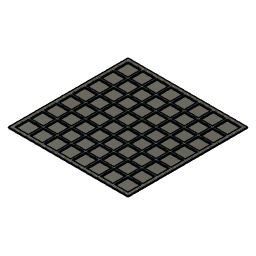
šachovnice v3 (Autodesk Fusion 360 design; units mm, degrees)
Autodesk Fusion 360 part; units mm, degrees
sketch "Sketch1" plane through (0, 0, 0) normal (0, 0, 1) x (1, 0, 0)
  line L0 (-133.2, 0) -> (133.2, 0)
  line L1 (133.2, 0) -> (133.2, -266.4)
  line L2 (133.2, -266.4) -> (-133.2, -266.4)
  line L3 (-133.2, -266.4) -> (-133.2, 0)
  line L4 (-100.2, 0) -> (-100.2, -266.4) construction
  line L5 (-133.2, -33.3) -> (133.2, -33.3) construction
  line L6 (-66.9, 0) -> (-66.9, -266.4) construction
  line L7 (-33.6, 0) -> (-33.6, -266.4) construction
  line L8 (-0.3, 0) -> (-0.3, -266.4) construction
  line L9 (33, 0) -> (33, -266.4) construction
  line L10 (66.3, 0) -> (66.3, -266.4) construction
  line L11 (99.6, 0) -> (99.6, -266.4) construction
  line L12 (-133.2, -66.6) -> (133.2, -66.6) construction
  line L13 (-133.2, -99.9) -> (133.2, -99.9) construction
  line L14 (-133.2, -133.2) -> (133.2, -133.2) construction
  line L15 (-133.2, -166.5) -> (133.2, -166.5) construction
  line L16 (-133.2, -199.8) -> (133.2, -199.8) construction
  line L17 (-133.2, -233.1) -> (133.2, -233.1) construction
  line L18 (-102.2, 0) -> (-102.2, -266.4)
  line L19 (-68.9, 0) -> (-68.9, -266.4)
  line L20 (-35.6, 0) -> (-35.6, -266.4)
  line L21 (-2.3, 0) -> (-2.3, -266.4)
  line L22 (31, 0) -> (31, -266.4)
  line L23 (64.3, 0) -> (64.3, -266.4)
  line L24 (97.6, 0) -> (97.6, -266.4)
  line L25 (-133.2, -35.3) -> (133.2, -35.3)
  line L26 (-133.2, -31.3) -> (133.2, -31.3)
  line L27 (-98.2, 0) -> (-98.2, -266.4)
  line L28 (-64.9, 0) -> (-64.9, -266.4)
  line L29 (-31.6, 0) -> (-31.6, -266.4)
  line L30 (1.7, 0) -> (1.7, -266.4)
  line L31 (35, 0) -> (35, -266.4)
  line L32 (68.3, 0) -> (68.3, -266.4)
  line L33 (101.6, 0) -> (101.6, -266.4)
  line L34 (-133.2, -64.6) -> (133.2, -64.6)
  line L35 (-133.2, -68.6) -> (133.2, -68.6)
  line L36 (-133.2, -97.9) -> (133.2, -97.9)
  line L37 (-133.2, -101.9) -> (133.2, -101.9)
  line L38 (-133.2, -131.2) -> (133.2, -131.2)
  line L39 (-133.2, -135.2) -> (133.2, -135.2)
  line L40 (-133.2, -164.5) -> (133.2, -164.5)
  line L41 (-133.2, -168.5) -> (133.2, -168.5)
  line L42 (-133.2, -197.8) -> (133.2, -197.8)
  line L43 (-133.2, -201.8) -> (133.2, -201.8)
  line L44 (-133.2, -231.1) -> (133.2, -231.1)
  line L45 (-133.2, -235.1) -> (133.2, -235.1)
  line L46 (137.2, -270.4) -> (-137.2, -270.4)
  line L47 (-137.2, -270.4) -> (-137.2, 4)
  line L48 (-137.2, 4) -> (137.2, 4)
  line L49 (137.2, 4) -> (137.2, -270.4)
  line L50 (-141.2, -274.4) -> (-141.2, 8)
  line L51 (-141.2, 8) -> (141.2, 8)
  line L52 (141.2, 8) -> (141.2, -274.4)
  line L53 (141.2, -274.4) -> (-141.2, -274.4)
  dimension "d1" = 266.4
  dimension "d8" = 33.3
  dimension "d9" = 0
  dimension "d10" = 33
  dimension "d11" = 33.3
  dimension "d14" = 0
  dimension "d15" = -33.3
  dimension "d16" = 2
  dimension "d17" = 2
  dimension "d18" = -2
  dimension "d19" = -2
  dimension "d20" = -4
  dimension "d21" = -8
  constraint horizontal L0
  constraint vertical L1
  constraint horizontal L2
  constraint vertical L3
  constraint equal L0 L3
  constraint midpoint origin L0
  constraint coincident L0 L4.start
  constraint coincident L2 L4.end
  constraint perpendicular L2 L4
  constraint coincident L3 L5.start
  constraint coincident L1 L5.end
  constraint perpendicular L1 L5
  measures "d1" distance of L0.start L0.end
  measures "d10" distance of L3 L4
  measures "d11" distance of L0 L5
extrude "Extrude1" add sketch "Sketch1" along normal blind 4 contours L0 L18 L26 L27 | L3 L18 L25 L26 | L18 L25 L26 L27 | L0 L19 L26 L28 | L19 L25 L26 L27 | L18 L25 L27 L34 | L3 L18 L34 L35 | L19 L25 L26 L28 | L18 L27 L34 L35 | L0 L20 L26 L29 | L20 L25 L26 L28 | L19 L25 L28 L34 | L19 L27 L34 L35 | L18 L27 L35 L36 | L3 L18 L36 L37 | L20 L25 L26 L29 | L19 L28 L34 L35 | L18 L27 L36 L37 | L0 L21 L26 L30 | L21 L25 L26 L29 | L20 L25 L29 L34 | L20 L28 L34 L35 | L19 L28 L35 L36 | L19 L27 L36 L37 | L18 L27 L37 L38 | L3 L18 L38 L39 | L21 L25 L26 L30 | L20 L29 L34 L35 | L19 L28 L36 L37 | L18 L27 L38 L39 | L0 L22 L26 L31 | L22 L25 L26 L30 | L21 L25 L30 L34 | L21 L29 L34 L35 | L20 L29 L35 L36 | L20 L28 L36 L37 | L19 L28 L37 L38 | L19 L27 L38 L39 | L18 L27 L39 L40 | L3 L18 L40 L41 | L22 L25 L26 L31 | L21 L30 L34 L35 | L20 L29 L36 L37 | L19 L28 L38 L39 | L18 L27 L40 L41 | L0 L23 L26 L32 | L23 L25 L26 L31 | L22 L25 L31 L34 | L22 L30 L34 L35 | L21 L30 L35 L36 | L21 L29 L36 L37 | L20 L29 L37 L38 | L20 L28 L38 L39 | L19 L28 L39 L40 | L19 L27 L40 L41 | L18 L27 L41 L42 | L3 L18 L42 L43 | L23 L25 L26 L32 | L22 L31 L34 L35 | L21 L30 L36 L37 | L20 L29 L38 L39 | L19 L28 L40 L41 | L18 L27 L42 L43 | L0 L24 L26 L33 | L24 L25 L26 L32 | L23 L25 L32 L34 | L23 L31 L34 L35 | L22 L31 L35 L36 | L22 L30 L36 L37 | L21 L30 L37 L38 | L21 L29 L38 L39 | L20 L29 L39 L40 | L20 L28 L40 L41 | L19 L28 L41 L42 | L19 L27 L42 L43 | L18 L27 L43 L44 | L3 L18 L44 L45 | L24 L25 L26 L33 | L23 L32 L34 L35 | L22 L31 L36 L37 | L21 L30 L38 L39 | L20 L29 L40 L41 | L19 L28 L42 L43 | L18 L27 L44 L45 | L1 L25 L26 L33 | L24 L25 L33 L34 | L24 L32 L34 L35 | L23 L32 L35 L36 | L23 L31 L36 L37 | L22 L31 L37 L38 | L22 L30 L38 L39 | L21 L30 L39 L40 | L21 L29 L40 L41 | L20 L29 L41 L42 | L20 L28 L42 L43 | L19 L28 L43 L44 | L19 L27 L44 L45 | L2 L18 L27 L45 | L24 L33 L34 L35 | L23 L32 L36 L37 | L22 L31 L38 L39 | L21 L30 L40 L41 | L20 L29 L42 L43 | L19 L28 L44 L45 | L1 L33 L34 L35 | L24 L33 L35 L36 | L24 L32 L36 L37 | L23 L32 L37 L38 | L23 L31 L38 L39 | L22 L31 L39 L40 | L22 L30 L40 L41 | L21 L30 L41 L42 | L21 L29 L42 L43 | L20 L29 L43 L44 | L20 L28 L44 L45 | L2 L19 L28 L45 | L24 L33 L36 L37 | L23 L32 L38 L39 | L22 L31 L40 L41 | L21 L30 L42 L43 | L20 L29 L44 L45 | L1 L33 L36 L37 | L24 L33 L37 L38 | L24 L32 L38 L39 | L23 L32 L39 L40 | L23 L31 L40 L41 | L22 L31 L41 L42 | L22 L30 L42 L43 | L21 L30 L43 L44 | L21 L29 L44 L45 | L2 L20 L29 L45 | L24 L33 L38 L39 | L23 L32 L40 L41 | L22 L31 L42 L43 | L21 L30 L44 L45 | L1 L33 L38 L39 | L24 L33 L39 L40 | L24 L32 L40 L41 | L23 L32 L41 L42 | L23 L31 L42 L43 | L22 L31 L43 L44 | L22 L30 L44 L45 | L2 L21 L30 L45 | L24 L33 L40 L41 | L23 L32 L42 L43 | L22 L31 L44 L45 | L1 L33 L40 L41 | L24 L33 L41 L42 | L24 L32 L42 L43 | L23 L32 L43 L44 | L23 L31 L44 L45 | L2 L22 L31 L45 | L24 L33 L42 L43 | L23 L32 L44 L45 | L1 L33 L42 L43 | L24 L33 L43 L44 | L24 L32 L44 L45 | L2 L23 L32 L45 | L24 L33 L44 L45 | L1 L33 L44 L45 | L2 L24 L33 L45 | L46 L47 L48 L49 | L50 L51 L52 L53
extrude "Extrude2" add sketch "Sketch1" along normal blind 1 contours L0 L3 L18 L26 | L0 L19 L26 L27 | L3 L18 L25 L34 | L0 L20 L26 L28 | L19 L25 L27 L34 | L3 L18 L35 L36 | L0 L21 L26 L29 | L20 L25 L28 L34 | L19 L27 L35 L36 | L3 L18 L37 L38 | L0 L22 L26 L30 | L21 L25 L29 L34 | L20 L28 L35 L36 | L19 L27 L37 L38 | L3 L18 L39 L40 | L0 L23 L26 L31 | L22 L25 L30 L34 | L21 L29 L35 L36 | L20 L28 L37 L38 | L19 L27 L39 L40 | L3 L18 L41 L42 | L0 L24 L26 L32 | L23 L25 L31 L34 | L22 L30 L35 L36 | L21 L29 L37 L38 | L20 L28 L39 L40 | L19 L27 L41 L42 | L3 L18 L43 L44 | L0 L1 L26 L33 | L24 L25 L32 L34 | L23 L31 L35 L36 | L22 L30 L37 L38 | L21 L29 L39 L40 | L20 L28 L41 L42 | L19 L27 L43 L44 | L2 L3 L18 L45 | L1 L25 L33 L34 | L24 L32 L35 L36 | L23 L31 L37 L38 | L22 L30 L39 L40 | L21 L29 L41 L42 | L20 L28 L43 L44 | L2 L19 L27 L45 | L1 L33 L35 L36 | L24 L32 L37 L38 | L23 L31 L39 L40 | L22 L30 L41 L42 | L21 L29 L43 L44 | L2 L20 L28 L45 | L1 L33 L37 L38 | L24 L32 L39 L40 | L23 L31 L41 L42 | L22 L30 L43 L44 | L2 L21 L29 L45 | L1 L33 L39 L40 | L24 L32 L41 L42 | L23 L31 L43 L44 | L2 L22 L30 L45 | L1 L33 L41 L42 | L24 L32 L43 L44 | L2 L23 L31 L45 | L1 L33 L43 L44 | L2 L24 L32 L45 | L1 L2 L33 L45
extrude "Extrude3" cut sketch "Sketch1" along normal blind 2 contours L50 L51 L52 L53
sketch "Sketch2" plane through (0, 0, 0) normal (0, 0, -1) x (1, 0, 0)
  line L0 (-137.2, 270.4) -> (-137.2, -4)
  line L1 (-137.2, -4) -> (137.2, -4)
  line L2 (137.2, -4) -> (137.2, 270.4)
  line L3 (137.2, 270.4) -> (-137.2, 270.4)
equation "d1 = ( 33.3 * 8 ) * 1 mm"
